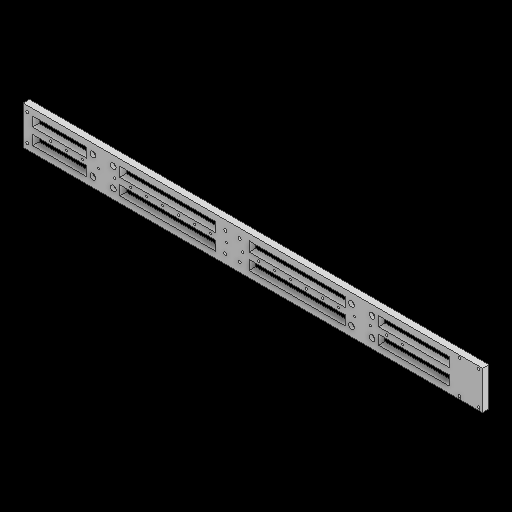
# Autodesk Inventor part: z_plate
Saved by Autodesk Inventor 2026.1 (Build 301233000, 233)
## iProperties
Created: 2025-09-27
Part Number: z_plate
Material: Generic
Document SubType Name: Modeling
Designer: drago
Density: 1 g/cm^3
Appearance: Default
Author: drago
Autodesk Inventor part; units mm, degrees
ref_plane "YZ Plane" through (0, 0, 0) normal (1, 0, 0) x (0, 1, 0)
ref_plane "XZ Plane" through (0, 0, 0) normal (0, 1, 0) x (-1, 0, 0)
ref_plane "XY Plane" through (0, 0, 0) normal (0, 0, 1) x (1, 0, 0)
sketch "Sketch1" plane through (0, 0, 0) normal (0, 0, 1) x (1, 0, 0)
  line L0 (-228.1805, 30) -> (228.1805, 30)
  line L1 (228.1805, 30) -> (228.1805, -30)
  line L2 (228.1805, -30) -> (-228.1805, -30)
  line L3 (-228.1805, -30) -> (-228.1805, 30)
  line L4 (0, 30) -> (0, -30) construction
  line L5 (-202.1805, 30) -> (-202.1805, -30) construction
  line L6 (202.1805, 30) -> (202.1805, -30) construction
  line L7 (-176.1805, 30) -> (-176.1805, -30)
  line L8 (176.1805, 30) -> (176.1805, -30)
  line L9 (228.1805, 0) -> (-228.1805, 0) construction
  line L10 (-26, 30) -> (-26, -30)
  line L11 (26, 30) -> (26, -30)
  line L12 (-228.1805, 30) -> (-327.25, 30)
  line L13 (-327.25, 30) -> (-327.25, -30)
  line L14 (-327.25, -30) -> (-228.1805, -30)
  line L15 (-312.25, 30) -> (-312.25, -30)
  line L16 (228.1805, 30) -> (390.75, 30)
  line L17 (390.75, 30) -> (390.75, -30)
  line L18 (390.75, -30) -> (228.1805, -30)
  line L19 (338.75, 30) -> (338.75, -30)
  line L20 (312.25, 30) -> (312.25, -30) construction
  line L21 (-312.25, 20) -> (-228.1805, 20)
  line L22 (-176.1805, 20) -> (-26, 20)
  line L23 (26, 20) -> (176.1805, 20)
  line L24 (228.1805, 20) -> (338.75, 20)
  line L25 (-312.25, -20) -> (-228.1805, -20)
  line L26 (-176.1805, -20) -> (-26, -20)
  line L27 (26, -20) -> (176.1805, -20)
  line L28 (228.1805, -20) -> (338.75, -20)
  line L29 (-312.25, 5) -> (-228.1805, 5)
  line L30 (-176.1805, 5) -> (-26, 5)
  line L31 (26, 5) -> (176.1805, 5)
  line L32 (228.1805, 5) -> (338.75, 5)
  line L33 (-312.25, -5) -> (-228.1805, -5)
  line L34 (-176.1805, -5) -> (-26, -5)
  line L35 (26, -5) -> (176.1805, -5)
  line L36 (228.1805, -5) -> (338.75, -5)
  line L37 (-228.1805, 0) -> (-327.25, 0) construction
  line L38 (228.1805, 0) -> (390.75, 0) construction
  line L39 (364.75, 30) -> (364.75, -30) construction
  line L40 (-319.75, 30) -> (-319.75, -30) construction
  circle A0 centre (384.75, 26) radius 2.15
  circle A1 centre (354.75, 26) radius 2.15
  circle A2 centre (354.75, -26) radius 2.15
  circle A3 centre (384.75, -26) radius 2.15
  circle A4 centre (-320.75, 21) radius 2.15
  circle A5 centre (-320.75, -21) radius 2.15
  circle A6 centre (-284.25, 0) radius 1.65
  circle A7 centre (-259.25, 0) radius 1.65
  circle A8 centre (-234.25, 0) radius 1.65
  circle A9 centre (-209.25, 0) radius 1.65
  circle A10 centre (-184.25, 0) radius 1.65
  circle A11 centre (-159.25, 0) radius 1.65
  circle A12 centre (-134.25, 0) radius 1.65
  circle A13 centre (-109.25, 0) radius 1.65
  circle A14 centre (-84.25, 0) radius 1.65
  circle A15 centre (-59.25, 0) radius 1.65
  circle A16 centre (-34.25, 0) radius 1.65
  circle A17 centre (-9.25, 0) radius 1.65
  circle A18 centre (15.75, 0) radius 1.65
  circle A19 centre (40.75, 0) radius 1.65
  circle A20 centre (65.75, 0) radius 1.65
  circle A21 centre (90.75, 0) radius 1.65
  circle A22 centre (115.75, 0) radius 1.65
  circle A23 centre (140.75, 0) radius 1.65
  circle A24 centre (165.75, 0) radius 1.65
  circle A25 centre (190.75, 0) radius 1.65
  circle A26 centre (215.75, 0) radius 1.65
  circle A27 centre (240.75, 0) radius 1.65
  circle A28 centre (265.75, 0) radius 1.65
  point P0 (0, 0)
  point P1 (0, 0)
  point P2 (-218.1805, 15)
  point P3 (-186.1805, 15)
  point P4 (-186.1805, -15)
  point P5 (-218.1805, -15)
  point P6 (186.1805, 15)
  point P7 (218.1805, 15)
  point P8 (218.1805, -15)
  point P9 (186.1805, -15)
  point P10 (-11, 16)
  point P11 (11, 16)
  point P12 (11, -16)
  point P13 (-11, -16)
  dimension "d39" = 404.361
  dimension "d42" = 52
  dimension "d43" = 30
  dimension "d44" = 32
  dimension "d45" = 32
  dimension "d46" = 30
  dimension "d52" = 52
  dimension "d53" = 15
  dimension "d54" = 60
  dimension "d56" = 52
  dimension "d57" = 78.5
  dimension "d59" = 718
  dimension "d60" = 10
  dimension "d61" = 10
  dimension "d62" = 10
  dimension "d74" = 4.3
  dimension "d75" = 4.3
  dimension "d76" = 4.3
  dimension "d77" = 4.3
  dimension "d78" = 4
  dimension "d79" = 6
  dimension "d80" = 30
  dimension "d81" = 4
  dimension "d82" = 4.3
  dimension "d83" = 6.5
  dimension "d84" = 9
  dimension "d85" = 4.3
  dimension "d93" = 32
  dimension "d94" = 22
  dimension "d95" = 3.3
  dimension "d96" = 43
  dimension "d99" = 25
  constraints: 78 end point, 55 point on line, 29 centre point, 15 perpendicular, 12 symmetric about line, 8 collinear, 8 vertical, 5 midpoint, 4 horizontal, 2 parallel, 1 coincident, 74 other
  measures "d39" distance between parallel lines of L6 L5
  measures "d42" distance between parallel lines of L11 L10
  measures "d43" distance of point (-186.18, -15) point (-186.18, 15)
  measures "d44" distance of point (-186.18, -15) point (-218.18, -15)
  measures "d45" distance of point (218.18, -15) point (186.18, -15)
  measures "d46" distance of point (218.18, -15) point (218.18, 15)
  measures "d52" distance between parallel lines of L7 L3
  measures "d53" distance between parallel lines of L15 L13
  measures "d54" distance of L16.end L17.end
  measures "d56" distance between parallel lines of L17 L19
  measures "d57" distance between parallel lines of L17 L20
  measures "d59" distance between parallel lines of L17 L13
  measures "d60" distance between parallel lines of L12 L21
  measures "d61" distance between parallel lines of L14 L25
  measures "d62" distance between parallel lines of L33 L29
  measures "d74" diameter of A0
  measures "d75" diameter of A1
  measures "d76" diameter of A2
  measures "d77" diameter of A3
  measures "d78" distance from line of L16 A0.centre
  measures "d79" distance from line of L17 A0.centre
  measures "d80" distance of A0.centre A1.centre
  measures "d81" distance from line of L16 A1.centre
  measures "d82" diameter of A4
  measures "d83" distance from line of L13 A4.centre
  measures "d84" distance from line of L12 A4.centre
  measures "d85" diameter of A5
  measures "d93" distance of point (11, -16) point (11, 16)
  measures "d94" distance of point (11, 16) point (-11, 16)
  measures "d95" diameter of A6
  measures "d96" distance from line of A6.centre L13
  measures "d99" distance of A6.centre A7.centre
extrude "Extrusion2" add sketch "Sketch1" against normal blind 10 contours L0 L7 L2 L3 | L3 L21 L15 L12 | L0 L10 L22 L7 | L15 L14 L13 L12 | L0 L11 L2 L10 | L3 L33 L15 L29 | L0 L8 L23 L11 | L30 L10 L34 L7 | L0 L1 L2 L8 | L3 L14 L15 L25 | L16 L19 L24 L1 | L31 L8 L35 L11 | L26 L10 L2 L7 | L16 L17 L18 L19 | L32 L19 L36 L1 | L27 L8 L2 L11 | L28 L19 L18 L1 | A0 | A1 | A2 | A3 | A4 | A5 | A6 | A7 | A8 | A9 | A10 | A11 | A12 | A13 | A14 | A15 | A16 | A17 | A18 | A19 | A20 | A21 | A22 | A23 | A24 | A25 | A26 | A27 | A28
hole "Hole2" at (-218.1805, 15, 0) at (-186.1805, 15, 0) at (-186.1805, -15, 0) at (-218.1805, -15, 0) at (186.1805, 15, 0) at (218.1805, 15, 0) at (218.1805, -15, 0) at (186.1805, -15, 0) direction (0, 0, -1) diameter 5.3 end through all counterbore diameter 9 counterbore depth 5
hole "Hole3" at (-320.75, 21, 0) at (-320.75, -21, 0) at (354.75, 26, 0) at (384.75, 26, 0) at (384.75, -26, 0) at (354.75, -26, 0) direction (0, 0, -1) diameter 4.3 end through all
hole "Hole4" at (-11, 16, 0) at (11, 16, 0) at (11, -16, 0) at (-11, -16, 0) direction (0, 0, -1) diameter 3.2 end through all counterbore diameter 5 counterbore depth 5
hole "Hole5" at (-284.25, 0, 0) at (-259.25, 0, 0) at (-234.25, 0, 0) at (-209.25, 0, 0) at (-184.25, 0, 0) at (-159.25, 0, 0) at (-134.25, 0, 0) at (-109.25, 0, 0) at (-84.25, 0, 0) at (-59.25, 0, 0) at (-34.25, 0, 0) at (15.75, 0, 0) at (-9.25, 0, 0) at (40.75, 0, 0) at (65.75, 0, 0) at (90.75, 0, 0) at (115.75, 0, 0) at (140.75, 0, 0) at (165.75, 0, 0) at (190.75, 0, 0) at (215.75, 0, 0) at (240.75, 0, 0) at (265.75, 0, 0) direction (0, 0, -1) diameter 3.3 end through all
equation "\"d39\" = dist_rails"
equation "\"d42\" = bracket_width"
equation "\"dist_rails\" = 404.361"
equation "\"bracket_width\" = 52"
body "Solid2"
